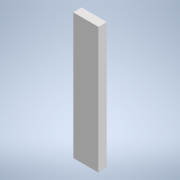
# Autodesk Inventor part: Part9
Saved by Autodesk Inventor 2020.2 (Build 242310000, 310)
## iProperties
Created: 2022-11-03
Part Number: Part9
Material: 一般
Document SubType Name: Modeling
Designer: Administrator
Density: 1 g/cm^3
Appearance: 既定
Author: Administrator
Autodesk Inventor part; units mm, degrees
ref_plane "YZ Plane" through (0, 0, 0) normal (1, 0, 0) x (0, 1, 0)
ref_plane "XZ Plane" through (0, 0, 0) normal (0, 1, 0) x (-1, 0, 0)
ref_plane "XY Plane" through (0, 0, 0) normal (0, 0, 1) x (1, 0, 0)
sketch "スケッチ1" plane through (0, 0, 0) normal (0, 1, 0) x (-1, 0, 0)
  line L0 (0, 0) -> (30, 0)
  line L1 (30, 0) -> (30, -10)
  line L2 (30, -10) -> (0, -10)
  line L3 (0, -10) -> (0, 0)
  dimension "d0" = 30
  dimension "d1" = 10
  constraints: 8 end point, 2 parallel, 1 horizontal, 1 perpendicular
  measures "d0" distance of L1.end L2.end
  measures "d1" distance of L0.end L1.end
extrude "押し出し1" add sketch "スケッチ1" along normal blind 200
